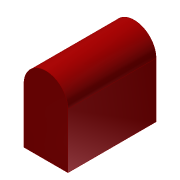
# Autodesk Inventor part: MSW-13-17_button#
Saved by Autodesk Inventor 2014 SP2 (Build 180247200, 247)
## iProperties
Company: ООО "Предприятие "Таврида Электрик Украина"
Created: 2022-06-28
Part Number: MSW-13-17_button#
Material: PC_ABS Plastic
Document SubType Name: Modeling
Designer: Воронежский
Mass: 0.00939027 g
Surface Area: 0.53708 cm^2
Volume: 0.0262832 cm^3
Density: 0.357273 g/cm^3
Appearance: Smooth - Red
TSKDver: 3.3.4.0
TSKD_DataStamp: 05.07.2022 15:26:07
Login: TAVRIDA\VPO
PCname: S-PC406
ESKDmaterialDescription: -
МатериалОбозначениеСтрокой: =<МатериалФорма> <МатериалРазмер>/<Material>
TEL_ID: -
Mass(g): =<Mass>
VLDS_FailCnt: 0
МатериалЕСКД: -
Author: Воронежский
Autodesk Inventor part; units mm, degrees
ref_plane "YZ Plane" through (0, 0, 0) normal (1, 0, 0) x (0, 1, 0)
ref_plane "XZ Plane" through (0, 0, 0) normal (0, 1, 0) x (-1, 0, 0)
ref_plane "XY Plane" through (0, 0, 0) normal (0, 0, 1) x (1, 0, 0)
sketch "Sketch2" plane through (0, 0, 0) normal (0, 0, 1) x (1, 0, 0)
  line L0 (-1, 2) -> (1, 2)
  line L1 (1, 2) -> (1, -2)
  line L2 (1, -2) -> (-1, -2)
  line L3 (-1, -2) -> (-1, 2)
  point P0 (0, 0)
  dimension "d2" = 4
  dimension "d3" = 2
  dimension "d4" = 1
  dimension "d5" = 2
  constraints: 8 end point, 2 parallel, 1 horizontal, 1 perpendicular
  measures "d2" distance of L2.end L0.start
  measures "d3" distance of L0.start L0.end
  measures "d4" distance from line of L1 point (0, 0)
  measures "d5" distance from line of L0 point (0, 0)
extrude "Extrusion1" add sketch "Sketch2" along normal blind 3.5
fillet "Fillet1" radius 1 2 edges at (1, 0, 3.5) (-1, 0, 3.5)
equation "\"d4\" = 0.5 * d3"
equation "\"d5\" = 0.5 * d2"
body "Solid1"
